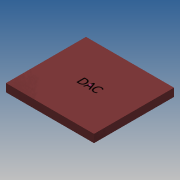
# Autodesk Inventor part: 17-0028-0014
Saved by Autodesk Inventor 2016 SP2 (Build 200236200, 236)
## iProperties
Created: 2017-10-26
Part Number: 17-0028-0014
Material: Generic
Document SubType Name: Modeling
Designer: Daan Giesen
Density: 0.001 g/cm^3
Appearance: Chestnut
Project: Digital PID Loop
Cost Center: 17-0028
User Status: Work in Progress
Authority: Reichsöllner, Lukas
RuleStatus: InUse
Category: IOP
Company: Universiteit van Amsterdam
BeforeDocSave0: Open Form
Author: Daan Giesen
Title: Digital PID Loop
Revision Number: A
Autodesk Inventor part; units mm, degrees
ref_plane "YZ Plane" through (0, 0, 0) normal (1, 0, 0) x (0, 1, 0)
ref_plane "XZ Plane" through (0, 0, 0) normal (0, 1, 0) x (-1, 0, 0)
ref_plane "XY Plane" through (0, 0, 0) normal (0, 0, 1) x (1, 0, 0)
sketch "Sketch1" plane through (0, 0, 0) normal (0, 0, 1) x (1, 0, 0)
  line L0 (0, 84) -> (0, -84) construction
  line L1 (-48.9937, 0) -> (48.8913, 0) construction
  line L2 (32.5, -60) -> (-32.5, -60)
  line L3 (-32.5, -60) -> (-32.5, 60)
  line L4 (-32.5, 60) -> (32.5, 60)
  line L5 (32.5, 60) -> (32.5, -60)
  line L6 (32.5, -60) -> (-32.5, 60) construction
  line L7 (-32.5, -60) -> (32.5, 60) construction
  point P0 (0, 0)
  dimension "d0" = 65
  dimension "d1" = 120
  constraints: 12 end point, 2 midpoint, 2 parallel, 1 horizontal, 1 perpendicular
  measures "d0" distance of L3.end L4.end
  measures "d1" distance of L2.end L3.end
extrude "Extrusion1" add sketch "Sketch1" along normal blind 10
sketch "Sketch2" plane through (0, 0, 10) normal (0, 0, 1) x (1, 0, 0)
  line L0 (-35.0101, 17.0569) -> (34.9078, 17.0569) construction
  line L1 (34.9078, 17.0569) -> (34.9078, -17.012) construction
  line L2 (34.9078, -17.012) -> (-35.0101, -17.012) construction
  line L3 (-35.0101, -17.012) -> (-35.0101, 17.0569) construction
  point P0 (0, 0)
  constraints: 2 other
body "Solid1"
